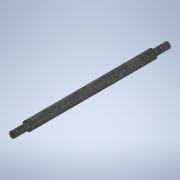
# Autodesk Inventor part: Eje.Proyecto 08
Saved by Autodesk Inventor 2021 (Build 250183000, 183)
## iProperties
Created: 2020-10-13
Part Number: Eje.Proyecto 08
Material: Steel
Document SubType Name: Modeling
Designer: CervMez
Density: 7.85 g/cm^3
Appearance: Plate
Mass: 20.617 g
Surface Area: 18.9124 cm^2
Volume: 2.62637 cm^3
Author: CervMez
Autodesk Inventor part; units mm, degrees
ref_plane "YZ Plane" through (0, 0, 0) normal (1, 0, 0) x (0, 1, 0)
ref_plane "XZ Plane" through (0, 0, 0) normal (0, 1, 0) x (-1, 0, 0)
ref_plane "XY Plane" through (0, 0, 0) normal (0, 0, 1) x (1, 0, 0)
sketch "Sketch1" plane through (0, 0, 0) normal (0, 0, 1) x (1, 0, 0)
  circle A0 centre (0, 0) radius 3
  dimension "d0" = 6
  constraints: 1 centre point, 1 coincident
  measures "d0" diameter of A0
extrude "Extrusion1" add sketch "Sketch1" against normal blind 84
sketch "Sketch2" plane through (0, 0, 0) normal (0, 0, 1) x (1, 0, 0)
  circle A0 centre (0, 0) radius 2
  circle A1 centre (0, 0) radius 3 projected
  dimension "d3" = 4
  constraints: 1 centre point, 1 coincident, 1 concentric
  measures "d3" diameter of A0
extrude "Extrusion2" add sketch "Sketch2" along normal blind 10 contours A0
sketch "Sketch3" plane through (0, 0, -84) normal (0, 0, -1) x (-1, 0, 0)
  circle A0 centre (0, 0) radius 2
  circle A1 centre (0, 0) radius 3 projected
  dimension "d6" = 4
  constraints: 1 centre point, 1 coincident, 1 concentric
  measures "d6" diameter of A0
extrude "Extrusion3" add sketch "Sketch3" along normal blind 10 contours A0
body "Solid1"
